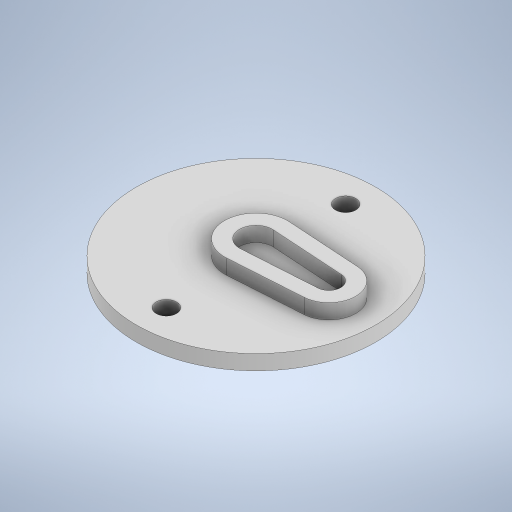
# Autodesk Inventor part: Thingy
Saved by Autodesk Inventor 2024 (Build 280153000, 153)
## iProperties
Created: 2023-04-23
Part Number: Thingy
Material: Generic
Document SubType Name: Modeling
Designer: byrne
Density: 1 g/cm^3
Appearance: Default
Author: byrne
Autodesk Inventor part; units mm, degrees
ref_plane "YZ Plane" through (0, 0, 0) normal (1, 0, 0) x (0, 1, 0)
ref_plane "XZ Plane" through (0, 0, 0) normal (0, 1, 0) x (-1, 0, 0)
ref_plane "XY Plane" through (0, 0, 0) normal (0, 0, 1) x (1, 0, 0)
sketch "Sketch1" plane through (0, 0, 0) normal (0, 1, 0) x (-1, 0, 0)
  circle A0 centre (0, 0) radius 25.4
  circle A1 centre (0, -19.05) radius 2.159
  circle A2 centre (0, 19.05) radius 2.159
  line L0 (0, 19.05) -> (0, -19.05)
  dimension "d0" = 50.8
  dimension "d1" = 4.318
  dimension "d2" = 4.318
  dimension "d3" = 38.1
  constraints: 3 centre point, 2 coincident, 2 end point, 1 midpoint, 1 vertical
  measures "d0" diameter of A0
  measures "d1" diameter of A1
  measures "d2" diameter of A2
  measures "d3" distance of L0.start L0.end
extrude "Extrusion1" add sketch "Sketch1" along normal blind 3.175
sketch "Sketch2" plane through (0, 3.175, 0) normal (0, 1, 0) x (1, 0, 0)
  arc A0 (0.2258, 3.4927) -> (0.2258, -3.4927) centre (0, 0) ccw
  arc A1 (15.6613, -2.4948) -> (15.6613, 2.4948) centre (15.5, 0) ccw
  line L0 (0.2258, 3.4927) -> (15.6613, 2.4948)
  line L1 (15.6613, -2.4948) -> (0.2258, -3.4927)
  line L2 (15.8661, 5.6632) -> (0.4306, 6.6611)
  arc A2 (0.4306, 6.6611) -> (0.4306, -6.6611) centre (0, 0) ccw
  line L3 (0.4306, -6.6611) -> (15.8661, -5.6632)
  arc A3 (15.8661, -5.6632) -> (15.8661, 5.6632) centre (15.5, 0) ccw
  dimension "d6" = 7
  dimension "d7" = 5
  dimension "d8" = 21.5
  dimension "d9" = 3.175
  constraints: 8 end point, 8 point on circle, 4 centre point, 4 tangent, 1 coincident, 1 horizontal alignment, 3 other
  measures "d6" diameter of A0
  measures "d7" diameter of A1
  measures "d9" distance between parallel lines of L0 L2
extrude "Extrusion2" add sketch "Sketch2" along normal blind 3.175
body "Solid1"
